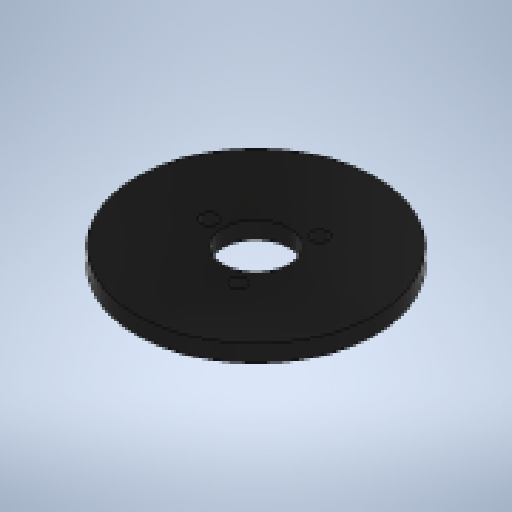
# Autodesk Inventor part: Interface Plate
Saved by Autodesk Inventor 2023 (Build 270158000, 158)
## iProperties
Created: 2022-07-31
Part Number: Interface Plate
Material: UHMW, Black
Document SubType Name: Modeling
Designer: Nathan Cai
Density: 0.94 g/cm^3
Appearance: Smooth - Black
Author: Nathan Cai
Autodesk Inventor part; units mm, degrees
ref_plane "YZ Plane" through (0, 0, 0) normal (1, 0, 0) x (0, 1, 0)
ref_plane "XZ Plane" through (0, 0, 0) normal (0, 1, 0) x (-1, 0, 0)
ref_plane "XY Plane" through (0, 0, 0) normal (0, 0, 1) x (1, 0, 0)
sketch "Sketch1" plane through (0, 0, 0) normal (0, 1, 0) x (-1, 0, 0)
  circle A0 centre (0, 0) radius 22.225
  circle A1 centre (0, 0) radius 6
  line L0 (0, 0) -> (22.225, 0) construction
  line L1 (8.6603, 0) -> (-4.3301, -7.5) construction
  line L2 (-4.3301, -7.5) -> (-4.3301, 7.5) construction
  line L3 (-4.3301, 7.5) -> (8.6603, 0) construction
  circle A2 centre (8.6603, 0) radius 1.5
  circle A3 centre (-4.3301, 7.5) radius 1.5
  circle A4 centre (-4.3301, -7.5) radius 1.5
  circle A5 centre (15.875, 0) radius 1.5
  circle A6 centre (11.2253, 11.2253) radius 1.5
  circle A7 centre (0, 15.875) radius 1.5
  circle A8 centre (-11.2253, 11.2253) radius 1.5
  circle A9 centre (-15.875, 0) radius 1.5
  circle A10 centre (-11.2253, -11.2253) radius 1.5
  circle A11 centre (0, -15.875) radius 1.5
  circle A12 centre (11.2253, -11.2253) radius 1.5
  dimension "d0" = 44.45
  dimension "d1" = 12
  dimension "d2" = 15
  dimension "d3" = 3
  dimension "d6" = 360
  dimension "d10" = 3
  dimension "d11" = 15.875
  dimension "d14" = 360
  constraints: 12 centre point, 8 end point, 4 coincident, 2 point on line, 1 horizontal, 1 horizontal alignment, 33 other
  measures "d1" diameter of A1
  measures "d2" distance of L1.end L2.end
  measures "d3" diameter of A2
  measures "d10" diameter of A5
  measures "d11" distance of point (0, 0) A5.centre
extrude "Extrusion1" add sketch "Sketch1" along normal blind 3.175
body "Solid1"
